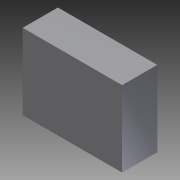
# Autodesk Inventor part: lid_f
Saved by Autodesk Inventor 2011 (Build 150239000, 239)
## iProperties
Created: 2011-05-24
Part Number: lid_f
Document SubType Name: Modeling
Designer: labuser
Density: 1 g/cm^3
Author: labuser
Autodesk Inventor part; units mm, degrees
ref_plane "YZ Plane" through (0, 0, 0) normal (1, 0, 0) x (0, 1, 0)
ref_plane "XZ Plane" through (0, 0, 0) normal (0, 1, 0) x (-1, 0, 0)
ref_plane "XY Plane" through (0, 0, 0) normal (0, 0, 1) x (1, 0, 0)
sketch "Sketch1" plane through (0, 0, 0) normal (0, 0, 1) x (1, 0, 0)
  line L0 (0, 0) -> (5.8, 0) construction
  line L1 (5.8, 0) -> (5.8, 4.3) construction
  line L2 (5.8, 4.3) -> (0, 4.3) construction
  line L3 (0, 4.3) -> (0, 0) construction
  line L4 (5.8, 4.3) -> (-5.5, 4.3)
  line L5 (-5.5, 4.3) -> (-5.5, -4.3)
  line L6 (-5.5, -4.3) -> (5.8, -4.3)
  line L7 (5.8, -4.3) -> (5.8, 4.3)
  dimension "d0" = 5.8
  dimension "d1" = 4.3
  dimension "d2" = 11.3
  dimension "d3" = 8.6
  constraints: 16 end point, 4 parallel, 2 horizontal, 2 perpendicular
  measures "d0" distance of L2.end L1.end
  measures "d1" distance of L1.end L0.end
  measures "d2" distance of L6.end L5.end
  measures "d3" distance of L5.end L4.end
extrude "Extrusion1" add sketch "Sketch1" along normal blind 4
body "Solid1"
